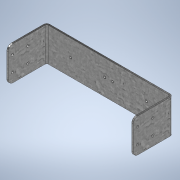
# Autodesk Inventor part: NEW Z Bracket
Saved by Autodesk Inventor 2022 (Build 260153000, 153)
## iProperties
Created: 2022-03-18
Part Number: NEW Z Bracket
Material: Generic
Document SubType Name: Sheet Metal
Designer: Nick
Density: 1 g/cm^3
Sheet Metal Rule: Default_mm
Appearance: Steel Galvanized
Flat Pattern Width: 4.4 cm
Flat Pattern Length: 26.2048 cm
Flat Pattern Area: 115.301 cm^2
Sheet Metal Width: 44.000 mm
Sheet Metal Length: 262.048 mm
Sheet Metal Area: 11530.103 mm^2
Author: Nick
Autodesk Inventor part; units mm, degrees
ref_plane "YZ Plane" through (0, 0, 0) normal (1, 0, 0) x (0, 1, 0)
ref_plane "XZ Plane" through (0, 0, 0) normal (0, 1, 0) x (-1, 0, 0)
ref_plane "XY Plane" through (0, 0, 0) normal (0, 0, 1) x (1, 0, 0)
sketch "Sketch1" plane through (0, 0, 0) normal (0, 0, 1) x (1, 0, 0)
  line L0 (0, 44) -> (161, 44)
  line L1 (161, 44) -> (161, 0)
  line L2 (161, 0) -> (0, 0)
  line L3 (0, 0) -> (0, 44)
  dimension "d0" = 161
  dimension "d1" = 44
  measures "d0" distance of L1.end L2.end
  measures "d1" distance of L0.end L1.end
extrude "Plate1" add sketch "Sketch1" along normal blind 2
sketch "Sketch2" plane through (0, 0, 2) normal (-1, 0, 0) x (0, -1, 0)
  line L0 (-44, 0) -> (0, 0)
  line L1 (0, 0) -> (0, 50)
  line L2 (0, 50) -> (-44, 50)
  line L3 (-44, 50) -> (-44, 0)
  constraints: 6 end point, 1 horizontal, 1 perpendicular, 1 vertical
edge flange "Flange1" height 52 angle 90 thickness 2 bend radius 2 thickness toward (-1, 0, 0) relief tear relief width 2 relief depth 1 corner gap 2 corner form 0 edges at (0, 22, 2) (161, 22, 2) wall of the first edge with corners at (0, 44, 2) (0, 0, 2) (0, 0, 52) (0, 44, 52)
bend "Bend1"
corner "Corner1"
sketch "Sketch3" plane through (163, 0, 52) normal (1, 0, 0) x (0, 0, -1)
  line L0 (0, 0) -> (0, 44) construction
  line L1 (5.5, 32) -> (5.5, 12) construction
  point P0 (52, 0)
  point P1 (25.5, 32)
  point P2 (25.5, 12)
  point P3 (0, 22)
  point P4 (5.5, 22)
  dimension "d13" = 20
  dimension "d14" = 20
  dimension "d15" = 5.5
  constraints: 3 horizontal alignment, 2 end point, 2 midpoint, 2 vertical alignment, 1 vertical
  measures "d13" distance of point (25.5, 32) L1.start
  measures "d14" distance of L1.end L1.start
  measures "d15" distance from line of L0 L1.start
hole "Hole1" at (163, 32, 46.5) at (163, 32, 26.5) at (163, 12, 46.5) at (163, 12, 26.5) direction (-1, 0, 0) diameter 3.4 end through all clearance for "Flat Head Machine Screw" size "M3" standard "Ansi Metric M Profile"
fillet "Corner Round1" radius 6 4 edges at (-1, 0, 52) (-1, 44, 52) (162, 0, 52) (162, 44, 52)
sketch "Sketch4" plane through (0, 0, 0) normal (0, 0, -1) x (-1, 0, 0)
  line L0 (-163, 0) -> (-163, 44) projected
  line L1 (2, 44) -> (2, 0) projected
  point P0 (0, 0)
  point P1 (-130, 22)
  point P2 (-85.5, 22)
  point P3 (-75.5, 22)
  point P4 (-31, 22)
  point P5 (-163, 22)
  dimension "d24" = 10
  dimension "d25" = 33
  dimension "d26" = 33
  dimension "d27" = 44.5
  dimension "d28" = 44.5
  constraints: 4 horizontal alignment, 1 midpoint
  measures "d24" distance of point (-75.5, 22) point (-85.5, 22)
  measures "d25" distance from line of L0 point (-130, 22)
  measures "d26" distance from line of L1 point (-31, 22)
  measures "d27" distance of point (-31, 22) point (-75.5, 22)
  measures "d28" distance of point (-130, 22) point (-85.5, 22)
hole "Hole2" at (130, 22, 0) at (85.5, 22, 0) at (75.5, 22, 0) at (31, 22, 0) direction (0, 0, 1) diameter 3.4 end through all clearance for "Flat Head Machine Screw" size "M3" standard "Ansi Metric M Profile"
equation "\"d21\" = Thickness"
equation "\"d2\" = Thickness"
equation "\"d3\" = BendReliefWidth"
equation "\"d4\" = BendReliefDepth"
equation "\"d5\" = MinimumRemnant"
equation "\"d6\" = TransitionRadius"
equation "\"d9\" = BendRadius"
equation "\"d10\" = CornerReliefSize"
equation "\"d11\" = GapSize"
equation "\"d12\" = JacobiRadiusSize"
equation "\"d26\" = d25"
equation "\"d28\" = d27"
equation "\"BendRadius\" = Thickness"
equation "\"BendReliefWidth\" = Thickness"
equation "\"BendReliefDepth\" = 0.5 * Thickness"
equation "\"CornerReliefSize\" = 4 * Thickness"
equation "\"MinimumRemnant\" = 2 * Thickness"
equation "\"TransitionRadius\" = BendRadius"
equation "\"JacobiRadiusSize\" = BendRadius"
equation "\"GapSize\" = Thickness"
equation "\"Thickness\" = 2"
body "Solid1"
